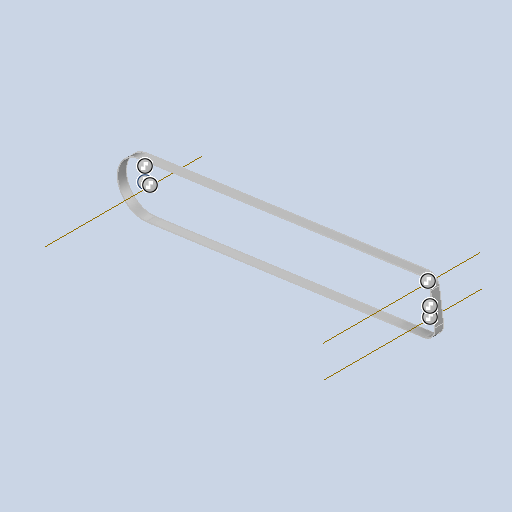
# Autodesk Inventor part: Pas synchroniczny
Saved by Autodesk Inventor 2023 (Build 270158000, 158)
## iProperties
CustomPartVersion: 1
Created: 2023-04-25
Part Number: Pas synchroniczny
Material: Rubber
Document SubType Name: Modeling
Designer: krzys
Density: 0.93 g/cm^3
Appearance: Rubber - Black - Version 1.1
Mass: 19.5672 g
Surface Area: 447.1 cm^2
Volume: 21.04 cm^3
Author: krzys
Autodesk Inventor part; units mm, degrees
sketch "Ścieżka szkicu" plane through (0, 0, 0) normal (0, 0, 1) x (1, 0, 0)
  arc A0 (3.3606, 47.2826) -> (16.5595, -47.2938) centre (10, 0) ccw
  arc A1 (543.3882, 105.4256) -> (523.6156, 120.337) centre (526.05, 103) ccw
  arc A2 (532.2226, 24.2268) -> (551.2284, 49.3843) centre (529.1616, 46.2972) ccw
  line L0 (532.2226, 24.2268) -> (16.5595, -47.2938)
  line L1 (3.3606, 47.2826) -> (523.6156, 120.337)
  line L2 (543.3882, 105.4256) -> (551.2284, 49.3843)
  constraints: 6 end point, 6 point on circle, 3 centre point
ref_plane "Płaszczyzna przekroju poprzecznego" through (16.5595, -47.2938, 0) normal (0.9905, 0.1374, 0) x (0, 0, 1)
ref_plane "Płaszczyzna konstrukcyjna2" through (10, 0, 0) normal (-1, 0, 0) x (0, 0, 1)
ref_plane "Płaszczyzna konstrukcyjna3" through (526.05, 103, 0) normal (-0.9979, -0.0651, 0) x (0, 0, 1)
ref_plane "Płaszczyzna konstrukcyjna4" through (529.1616, 46.2972, 0) normal (-0.04, 0.9992, 0) x (0, 0, 1)
sketch "Przekrój poprzeczny" plane through (16.5595, -47.2938, 0) normal (0.9905, 0.1374, 0) x (0, 0, 1)
  line L0 (-8, 0.5) -> (8, 0.5)
  line L1 (8, 0.5) -> (8, -0.5)
  line L2 (8, -0.5) -> (-8, -0.5)
  line L3 (-8, -0.5) -> (-8, 0.5)
  line L4 (-8, 0) -> (8, 0) construction
  point P0 (0, 0)
  point P1 (0, 0)
  dimension "d0" = 16
  dimension "d4" = 0.5
  dimension "d5" = 0.5
  constraints: 10 end point, 3 midpoint, 2 parallel, 1 coincident, 1 horizontal, 1 perpendicular, 1 other
  measures "d0" distance between parallel lines of L1 L3
  measures "d4" distance between parallel lines of L2 L4
  measures "d5" distance between parallel lines of L4 L0
sweep "Pas" add profiles "Przekrój poprzeczny" path "Ścieżka szkicu"
equation "\"d0\" = da_B"
equation "\"d4\" = da_a"
equation "\"d5\" = da_a2"
equation "\"da_B\" = 16"
equation "\"da_pb\" = 5"
equation "\"da_L\" = 1315"
equation "\"da_a\" = 0.5"
equation "\"da_S\" = 2.65"
equation "\"da_Beta\" = 20deg"
equation "\"da_Ht\" = 1.2"
equation "\"da_H\" = 2.2"
equation "\"da_a2\" = 0.5"
body "Solid1"
